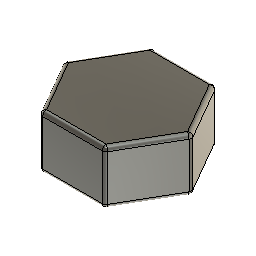
Gas can cap (Autodesk Fusion 360 design; units mm, degrees)
Autodesk Fusion 360 part; units mm, degrees
note: some values were not read from the file. Set by a fixed rule: which sketch regions a step uses.
sketch "Sketch1" plane through (0, 0, 0) normal (0, 0, 1) x (1, 0, 0)
  circle A0 centre (0, 0) radius 11
  circle A1 centre (0, 0) radius 9.5 construction
  line L0 (8.0829, 14) -> (-8.0829, 14)
  line L1 (-8.0829, 14) -> (-16.1658, 0)
  line L2 (-16.1658, 0) -> (-8.0829, -14)
  line L3 (-8.0829, -14) -> (8.0829, -14)
  line L4 (8.0829, -14) -> (16.1658, 0)
  line L5 (16.1658, 0) -> (8.0829, 14)
  dimension "d1" = 22
  dimension "d2" = 19
  dimension "d3" = 14
  constraint coincident A0.centre A1.centre
  constraint concentric A0 A1
  constraint horizontal L0
  measures "d1" diameter of A0
  measures "d2" diameter of A1
  measures "d3" distance of A0.centre L3
extrude "Extrude1" add sketch "Sketch1" along normal blind 13.5 contours A0 | L0 L1 L2 L3 L4 L5
extrude "Extrude2" cut sketch "Sketch1" along normal blind 10.5 contours A0
ref_plane "WorkPlane1" through (0, 0, 1.2) normal (0, 0, 1) x (1, 0, 0)
coil "CoilPrimitive1" add diameter 22 section triangle in size 2 inside turns 2 pitch 4 right hand placed x (1, 0, 0) y (0, 1, 0) z (0, 0, 1) at (0, 0, 1.2)
chamfer "Chamfer1" distance 3 distance2 1 2 edges at (10, 0, 0.6226) (10, 0, 1.7774) measured on face at (-8.7793, 5.4499, 2.0765) measured on face at (-7.9768, 6.5686, 3.5312)
chamfer "Chamfer2" distance 0.2 angle 45 1 edges at (-10.2556, -3.9778, 0)
fillet "Fillet1" radius 1 6 faces at (-2.6943, -14, 4.5) (-13.4715, -4.6667, 4.5) (2.6943, 14, 4.5) (-10.7772, 9.3333, 4.5) (10.1809, 10.3662, 6.0552) (10.7559, -9.3702, 5.8641)
chamfer "Chamfer3" distance 1 distance2 3 2 edges at (10, 0, 8.6226) (10, 0, 9.7774) measured on face at (10.3333, 0, 9.2) measured on face at (10.3333, 0, 9.2)
sketch "Sketch4" plane through (0, 0, 0) normal (0, 0, -1) x (1, 0, 0)
  circle A0 centre (0, 0) radius 11.2
  line L0 (-7.5056, -13) -> (7.5056, -13)
  line L1 (7.5056, -13) -> (15.0111, 0)
  line L2 (15.0111, 0) -> (7.5056, 13)
  line L3 (7.5056, 13) -> (-7.5056, 13)
  line L4 (-7.5056, 13) -> (-15.0111, 0)
  line L5 (-15.0111, 0) -> (-7.5056, -13)
  spline S0 degree 3 poles (8.4856, -2.9992) (7.7072, -5.2013) (6.0356, -7.073) (3.935, -8.0942) (1.8381, -9.1136) (-0.6612, -9.2736) (-2.8709, -8.5298) (-5.077, -7.7873) (-6.9685, -6.1529) (-8.0231, -4.0779) (-9.0762, -2.0061) (-9.2828, 0.4808) (-8.5861, 2.698) (-7.8903, 4.9122) (-6.3019, 6.8317) (-4.2571, 7.9295) (-2.2149, 9.0259) (0.2589, 9.2901) (2.4866, 8.6497) (4.7117, 8.01) (6.6656, 6.4753) (7.8143, 4.4651) (9.0166, 2.3609) (9.3175, -0.2391) (8.6275, -2.5623) (7.9635, -4.7983) (6.3929, -6.7507) (4.351, -7.8784) (2.3157, -9.0024) (-0.1637, -9.294) (-2.4042, -8.6729) (-4.6386, -8.0536) (-6.6095, -6.5338) (-7.7766, -4.5304) (-8.9411, -2.5314) (-9.2923, -0.074) (-8.7342, 2.1711) (-8.1728, 4.4296) (-6.6974, 6.4468) (-4.7151, 7.666) (-2.7434, 8.8788) (-0.2931, 9.2883) (1.9658, 8.7827) (4.2281, 8.2763) (6.2724, 6.8579) (7.5387, 4.9161) (7.9289, 4.3177) (8.2475, 3.6727) (8.4856, 2.9992) knots 0.339741 0.339741 0.339741 0.339741 1.118291 1.118291 1.118291 1.89546 1.89546 1.89546 2.67135 2.67135 2.67135 3.446058 3.446058 3.446058 4.219682 4.219682 4.219682 4.992317 4.992317 4.992317 5.764059 5.764059 5.764059 6.57188 6.57188 6.57188 7.349397 7.349397 7.349397 8.124399 8.124399 8.124399 8.897278 8.897278 8.897278 9.668414 9.668414 9.668414 10.444148 10.444148 10.444148 11.215776 11.215776 11.215776 11.988509 11.988509 11.988509 12.22663 12.22663 12.22663 12.22663
  circle A1 centre (0, 0) radius 9.7
  dimension "d22" = 19.4
  constraint concentric A0 A1
  measures "d22" diameter of A1
extrude "Extrude3" cut sketch "Sketch4" against normal blind 10.5 contours A1
equation "d3 = d1 / 2 + 3 mm"
named bodies: "Gas can cap"
